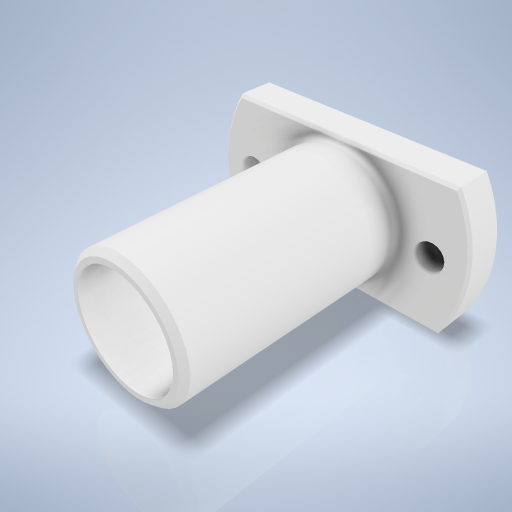
# Autodesk Inventor part: 11
Saved by Autodesk Inventor 2024.2 (Build 282272000, 272)
## iProperties
Created: 2024-05-14
Part Number: 11
Material: Acetalharz, Weiß
Document SubType Name: Modeling
Designer: Fabri
Density: 1.425 g/cm^3
Appearance: Glatt - Weiß
Author: Fabri
Autodesk Inventor part; units mm, degrees
ref_plane "YZ Plane" through (0, 0, 0) normal (1, 0, 0) x (0, 1, 0)
ref_plane "XZ Plane" through (0, 0, 0) normal (0, 1, 0) x (-1, 0, 0)
ref_plane "XY Plane" through (0, 0, 0) normal (0, 0, 1) x (1, 0, 0)
sketch "Skizze1" plane through (0, 0, 0) normal (0, 1, 0) x (-1, 0, 0)
  circle A0 centre (0, 0) radius 24
  dimension "d0" = 48
  constraints: 1 centre point, 1 coincident
  measures "d0" diameter of A0
extrude "Extrusion1" add sketch "Skizze1" along normal blind 6.5
sketch "Skizze2" plane through (0, 6.5, 0) normal (0, 1, 0) x (1, 0, 0)
  circle A0 centre (0, 0) radius 24 projected
  line L0 (-20.4878, -12.5) -> (20.4878, -12.5)
  circle A1 centre (0, 0) radius 24 projected
  line L1 (-20.4878, 12.5) -> (20.4878, 12.5)
  line L2 (-24, 0) -> (24, 0) construction
  dimension "d3" = 12.5
  dimension "d4" = 12.5
  constraints: 6 end point, 6 point on circle, 2 parallel, 1 horizontal, 1 other
  measures "d3" distance from line of point (0, 0) L0
  measures "d4" distance from line of L1 point (0, 0)
extrude "Extrusion2" cut sketch "Skizze2" against normal up to surface (6.5 mm away) contours L1 A0 | A0 L0
sketch "Skizze3" plane through (0, 0, 0) normal (0, -1, 0) x (1, 0, 0)
  circle A0 centre (0, 0) radius 11.5
  dimension "d7" = 23
  constraints: 1 centre point, 1 coincident
  measures "d7" diameter of A0
extrude "Extrusion3" add sketch "Skizze3" along normal blind 40.5
sketch "Skizze4" plane through (0, 6.5, 0) normal (0, 1, 0) x (1, 0, 0)
  point P0 (0, 0)
  point P1 (0, 0)
  constraints: 1 coincident
hole "Bohrung1" at (0, 6.5, 0) direction (0, -1, 0) diameter 19 depth 47
sketch "Skizze5" plane through (0, 6.5, 0) normal (0, 1, 0) x (1, 0, 0)
  line L0 (-20.4878, -12.5) -> (20.4878, -12.5) projected
  point P0 (0, 0)
  point P1 (17.5, 0)
  point P2 (-17.5, 0)
  dimension "d25" = 12.5
  dimension "d26" = 12.5
  dimension "d27" = 17.5
  dimension "d28" = 17.5
  constraints: 2 horizontal alignment
  measures "d25" distance from line of L0 point (17.5, 0)
  measures "d26" distance from line of L0 point (-17.5, 0)
  measures "d27" distance of point (0, 0) point (17.5, 0)
  measures "d28" distance of point (0, 0) point (-17.5, 0)
hole "Bohrung2" at (17.5, 6.5, 0) at (-17.5, 6.5, 0) direction (0, -1, 0) diameter 5 depth 6.5
fillet "Rundung1" radius 1 1 edges at (-11.5, 0, 0)
chamfer "Fasen1" distance 1 angle 45 1 edges at (-11.5, -40.5, 0)
chamfer "Fasen2" distance 0.5 angle 45 4 edges at (0, 0, -12.5) (-24, 0, 0) (24, 0, 0) (0, 0, 12.5)
